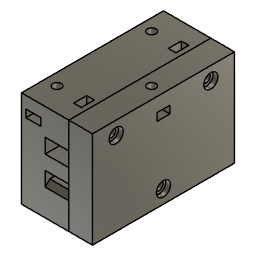
y-belt-holder (Autodesk Fusion 360 design; units mm, degrees)
Autodesk Fusion 360 part; units mm, degrees
sketch "main" plane through (0, 0, 0) normal (1, 0, 0) x (0, 1, 0)
  line L0 (0, 0) -> (60, 0)
  line L1 (60, 0) -> (60, -18.1)
  line L2 (60, -18.1) -> (0, -18.1)
  line L3 (0, -18.1) -> (0, 0)
  line L4 (0, 0) -> (60, 0)
  line L5 (60, 0) -> (60, 17.4)
  line L6 (60, 17.4) -> (0, 17.4)
  line L7 (0, 17.4) -> (0, 0)
  line L8 (0, 17.4) -> (60, 17.4)
  line L9 (60, 17.4) -> (60, 6.15)
  line L10 (60, 6.15) -> (0, 6.15)
  line L11 (0, 6.15) -> (0, 17.4)
  line L12 (0, -18.1) -> (10, -18.1) construction
  line L13 (10, -18.1) -> (10, 0) construction
  line L14 (10, 0) -> (0, 0) construction
  line L15 (0, 0) -> (0, -18.1) construction
  line L16 (60, -18.1) -> (50, -18.1) construction
  line L17 (50, -18.1) -> (50, 0) construction
  line L18 (50, 0) -> (60, 0) construction
  line L19 (60, 0) -> (60, -18.1) construction
  line L20 (10, 0) -> (18, 0)
  line L21 (18, 0) -> (18, -8)
  line L22 (18, -8) -> (10, -8)
  line L23 (10, -8) -> (10, 0)
  line L24 (10, -18.1) -> (18, -18.1)
  line L25 (18, -18.1) -> (18, -10.1)
  line L26 (18, -10.1) -> (10, -10.1)
  line L27 (10, -10.1) -> (10, -18.1)
  line L28 (50, -18.1) -> (42, -18.1)
  line L29 (42, -18.1) -> (42, -10.1)
  line L30 (42, -10.1) -> (50, -10.1)
  line L31 (50, -10.1) -> (50, -18.1)
  line L32 (50, 0) -> (42, 0)
  line L33 (42, 0) -> (42, -8)
  line L34 (42, -8) -> (50, -8)
  line L35 (50, -8) -> (50, 0)
  line L36 (10, 0) -> (18, -8) construction
  line L37 (18, 0) -> (10, -8) construction
  line L38 (42, 0) -> (50, -8) construction
  line L39 (50, 0) -> (42, -8) construction
  line L40 (14, -4) -> (25, -4) construction
  line L41 (46, -4) -> (35, -4) construction
  circle A0 centre (25, -4) radius 4
  circle A1 centre (35, -4) radius 4
  line L42 (0, -10.1) -> (60, -10.1)
  line L43 (0, -8) -> (60, -8)
  dimension "d1" = 60
  dimension "d2" = 18.1
  dimension "d3" = 60
  dimension "d4" = 17.4
  dimension "d5" = 60
  dimension "d6" = 11.25
  dimension "d7" = 10
  dimension "d8" = 18.1
  dimension "d9" = 10
  dimension "d10" = 18.1
  dimension "d11" = 8
  dimension "d12" = 8
  dimension "d13" = 8
  dimension "d14" = 8
  dimension "d15" = 8
  dimension "d16" = 8
  dimension "d17" = 8
  dimension "d18" = 8
  dimension "d19" = 11
  dimension "d20" = 11
  dimension "d21" = 8
  dimension "d22" = 8
  constraint horizontal L0
  constraint vertical L1
  constraint horizontal L2
  constraint vertical L3
  constraint coincident L0.start L3.end
  constraint horizontal L4
  constraint vertical L5
  constraint horizontal L6
  constraint vertical L7
  constraint horizontal L8
  constraint vertical L9
  constraint horizontal L10
  constraint vertical L11
  constraint horizontal L12
  constraint vertical L13
  constraint horizontal L14
  constraint vertical L15
  constraint horizontal L16
  constraint vertical L17
  constraint horizontal L18
  constraint vertical L19
  constraint horizontal L20
  constraint vertical L21
  constraint horizontal L22
  constraint vertical L23
  constraint horizontal L24
  constraint vertical L25
  constraint horizontal L26
  constraint vertical L27
  constraint horizontal L28
  constraint vertical L29
  constraint horizontal L30
  constraint vertical L31
  constraint horizontal L32
  constraint vertical L33
  constraint horizontal L34
  constraint vertical L35
  constraint midpoint L36 L40.start
  constraint perpendicular L21 L40
  constraint midpoint L38 L41.start
  constraint horizontal L41
  constraint coincident L40.end A0.centre
  constraint coincident L41.end A1.centre
  constraint coincident L3 L42.start
  constraint coincident L19 L42.end
  constraint perpendicular L19 L42
  constraint coincident L3 L43.start
  constraint coincident L19 L43.end
  constraint perpendicular L19 L43
  measures "d1" distance of L0.start L0.end
  measures "d2" distance of L0.start L2.end
  measures "d3" distance of L0.start L0.end
  measures "d4" distance of L0.start L6.end
  measures "d5" distance of L6.end L5.end
  measures "d6" distance of L6.end L10.end
  measures "d7" distance of L2.end L12.end
  measures "d8" distance of L2.end L0.start
  measures "d9" distance of L1.end L16.end
  measures "d10" distance of L1.end L0.end
  measures "d11" distance of L13.end L20.end
  measures "d12" distance of L13.end L22.end
  measures "d13" distance of L12.end L24.end
  measures "d14" distance of L12.end L26.end
  measures "d15" distance of L16.end L28.end
  measures "d16" distance of L16.end L30.end
  measures "d17" distance of L17.end L32.end
  measures "d18" distance of L17.end L34.end
  measures "d19" distance of L40.start L40.end
  measures "d20" distance of L41.start L41.end
  measures "d21" diameter of A0
  measures "d22" diameter of A1
extrude "Extrude1" add sketch "main" against normal blind 10 makes body 1
extrude "Extrude2" add sketch "main" along normal blind 10 contours L0 L3 L4 L23 L43 | L0 L4 L20 L21 L22 L23 L43 | L5 L6 L7 L8 L9 L10 L11 | L2 L3 L27 L42 | A0 | L2 L24 L25 L26 L27 L42 | L0 L1 L4 L35 L43 | A1 | L2 L25 L29 L42 | L0 L4 L32 L33 L34 L35 L43 | L2 L28 L29 L30 L31 L42 | L1 L2 L31 L42 bodies 1
chamfer "Chamfer2" distance 2 angle 45 9 edges at (5, 0, -8) (5, 18, -8) (10, 9, -8) (10, 30, -10.1) (5, 0, -10.1) (10, 51, -8) (5, 60, -8) (5, 60, -10.1) (5, 42, -8) on bodies 1
chamfer "Chamfer3" distance 1 angle 45 2 edges at (10, 21.2707, -5.4465) (10, 31.2707, -5.4465) on bodies 1
sketch "main-top-mount" plane through (0, 0, 17.4) normal (0, 0, 1) x (-1, 0, 0)
  line L0 (-10, -60) -> (10, -60)
  line L1 (10, -60) -> (10, 0)
  line L2 (10, 0) -> (-10, 0)
  line L3 (-10, 0) -> (-10, -60)
  line L4 (10, 0) -> (0, 0) construction
  line L5 (0, 0) -> (0, -20) construction
  line L6 (0, -20) -> (10, -20) construction
  line L7 (10, -20) -> (10, 0) construction
  line L8 (10, -60) -> (0, -60) construction
  line L9 (0, -60) -> (0, -40) construction
  line L10 (0, -40) -> (10, -40) construction
  line L11 (10, -40) -> (10, -60) construction
  line L12 (10, 0) -> (0, -20) construction
  line L13 (0, 0) -> (10, -20) construction
  line L14 (10, -60) -> (0, -40) construction
  line L15 (0, -60) -> (10, -40) construction
  circle A0 centre (5, -10) radius 1.8
  circle A1 centre (5, -50) radius 1.8
  line L16 (6.5733, -12.725) -> (8.1466, -10)
  line L17 (8.1466, -10) -> (6.5733, -7.275)
  line L18 (6.5733, -7.275) -> (3.4267, -7.275)
  line L19 (3.4267, -7.275) -> (1.8534, -10)
  line L20 (1.8534, -10) -> (3.4267, -12.725)
  line L21 (3.4267, -12.725) -> (6.5733, -12.725)
  line L22 (6.5733, -52.725) -> (8.1466, -50)
  line L23 (8.1466, -50) -> (6.5733, -47.275)
  line L24 (6.5733, -47.275) -> (3.4267, -47.275)
  line L25 (3.4267, -47.275) -> (1.8534, -50)
  line L26 (1.8534, -50) -> (3.4267, -52.725)
  line L27 (3.4267, -52.725) -> (6.5733, -52.725)
  line L28 (8.1466, -10) -> (8.1466, 0)
  line L29 (1.8534, -10) -> (1.8534, 0)
  line L30 (1.8534, -50) -> (1.8534, -60)
  line L31 (8.1466, -50) -> (8.1466, -60)
  point P0 (5, -10)
  point P1 (5, -50)
  dimension "d32" = 10
  dimension "d33" = 20
  dimension "d34" = 10
  dimension "d35" = 20
  dimension "d36" = 3.6
  dimension "d37" = 3.6
  dimension "d38" = 2.725
  dimension "d39" = 2.725
  dimension "d40" = 10
  dimension "d41" = 10
  dimension "d42" = 10
  dimension "d43" = 10
  constraint horizontal L4
  constraint vertical L5
  constraint horizontal L6
  constraint vertical L7
  constraint coincident L1.end L2.start
  constraint horizontal L8
  constraint vertical L9
  constraint horizontal L10
  constraint vertical L11
  constraint coincident L0.end L1.start
  constraint coincident L4.end L5.start
  constraint midpoint L13 P0
  constraint midpoint L15 P1
  constraint coincident P0 A0.centre
  constraint coincident P1 A1.centre
  constraint vertical L28
  constraint vertical L29
  constraint vertical L30
  constraint vertical L31
  measures "d32" distance of L1.end L4.end
  measures "d33" distance of L1.end L6.end
  measures "d34" distance of L0.end L8.end
  measures "d35" distance of L0.end L10.end
  measures "d36" diameter of A0
  measures "d37" diameter of A1
  measures "d38" distance of P0 L21
  measures "d39" distance of P1 L27
  measures "d40" distance of L16.end L28.end
  measures "d41" distance of L19.end L29.end
  measures "d42" distance of L25.end L30.end
  measures "d43" distance of L22.end L31.end
extrude "Extrude3" cut sketch "main-top-mount" against normal blind 16 contours A0 | A1 bodies 1
extrude "Extrude4" cut sketch "main-top-mount" against normal blind 3.2 from surface at -5 contours L0 L22 L26 L27 L30 L31 | L22 L23 L24 L25 L26 L27 | L2 L17 L18 L19 L28 L29 | L16 L17 L18 L19 L20 L21 bodies 1
extrude "Extrude5" add 1 faces at (3.3333, 40, -18.1) along direction (0, 0, -1) blind 5.25 on bodies 1 bodies 1
sketch "cover" plane through (0, 0, 0) normal (0, 1, 0) x (1, 0, 0)
  line L0 (0, 23.35) -> (10, 23.35) construction
  line L1 (10, 23.35) -> (10, -17.4) construction
  line L2 (10, -17.4) -> (0, -17.4) construction
  line L3 (0, -17.4) -> (0, 23.35) construction
  line L4 (-10, 23.35) -> (10, 23.35) construction
  line L5 (-10, -17.4) -> (10, -17.4) construction
  line L6 (10, 23.35) -> (20, 23.35)
  line L7 (20, 23.35) -> (20, -17.4)
  line L8 (20, -17.4) -> (10, -17.4)
  line L9 (10, -17.4) -> (10, 23.35)
  dimension "d51" = 10
  dimension "d52" = 10
  constraint horizontal L0
  constraint vertical L1
  constraint horizontal L2
  constraint vertical L3
  constraint coincident L1.end L5
  constraint midpoint L0.start L4
  constraint horizontal L6
  constraint vertical L7
  constraint horizontal L8
  constraint vertical L9
  constraint coincident L0.end L1.start
  measures "d51" distance of L0.start L0.end
  measures "d52" distance of L0.end L6.end
extrude "Extrude6" add sketch "cover" along normal blind 60 separate body makes body 2
sketch "cover-joint" plane through (10, 0, 0) normal (1, 0, 0) x (0, 1, 0)
  line L0 (0, 6.15) -> (60, 6.15)
  line L1 (60, 6.15) -> (60, 17.4)
  line L2 (60, 17.4) -> (0, 17.4)
  line L3 (0, 17.4) -> (0, 6.15)
  line L4 (0, 17.4) -> (20, 17.4) construction
  line L5 (20, 17.4) -> (20, 6.15) construction
  line L6 (20, 6.15) -> (0, 6.15) construction
  line L7 (0, 6.15) -> (0, 17.4) construction
  line L8 (60, 17.4) -> (40, 17.4) construction
  line L9 (40, 17.4) -> (40, 6.15) construction
  line L10 (40, 6.15) -> (60, 6.15) construction
  line L11 (60, 6.15) -> (60, 17.4) construction
  line L12 (0, 6.15) -> (60, 6.15) construction
  line L13 (60, 6.15) -> (60, -12.1) construction
  line L14 (60, -12.1) -> (0, -12.1) construction
  line L15 (0, -12.1) -> (0, 6.15) construction
  line L16 (0, -12.1) -> (60, -12.1) construction
  line L17 (60, -12.1) -> (60, -23.35) construction
  line L18 (60, -23.35) -> (0, -23.35) construction
  line L19 (0, -23.35) -> (0, -12.1) construction
  line L20 (0, -12.1) -> (60, -23.35) construction
  line L21 (60, -12.1) -> (0, -23.35) construction
  line L22 (0, 17.4) -> (20, 6.15) construction
  line L23 (20, 17.4) -> (0, 6.15) construction
  line L24 (40, 17.4) -> (60, 6.15) construction
  line L25 (60, 17.4) -> (40, 6.15) construction
  circle A0 centre (10, 11.775) radius 1.8
  circle A1 centre (50, 11.775) radius 1.8
  circle A2 centre (30, -17.725) radius 1.8
  line L26 (32.725, -16.1517) -> (30, -14.5784)
  line L27 (30, -14.5784) -> (27.275, -16.1517)
  line L28 (27.275, -16.1517) -> (27.275, -19.2983)
  line L29 (27.275, -19.2983) -> (30, -20.8716)
  line L30 (30, -20.8716) -> (32.725, -19.2983)
  line L31 (32.725, -19.2983) -> (32.725, -16.1517)
  line L32 (12.725, 13.3483) -> (10, 14.9216)
  line L33 (10, 14.9216) -> (7.275, 13.3483)
  line L34 (7.275, 13.3483) -> (7.275, 10.2017)
  line L35 (7.275, 10.2017) -> (10, 8.6284)
  line L36 (10, 8.6284) -> (12.725, 10.2017)
  line L37 (12.725, 10.2017) -> (12.725, 13.3483)
  line L38 (52.725, 13.3483) -> (50, 14.9216)
  line L39 (50, 14.9216) -> (47.275, 13.3483)
  line L40 (47.275, 13.3483) -> (47.275, 10.2017)
  line L41 (47.275, 10.2017) -> (50, 8.6284)
  line L42 (50, 8.6284) -> (52.725, 10.2017)
  line L43 (52.725, 10.2017) -> (52.725, 13.3483)
  line L44 (7.275, 13.3483) -> (7.275, 17.4)
  line L45 (12.725, 13.3483) -> (12.725, 17.4)
  line L46 (47.275, 13.3483) -> (47.275, 17.4)
  line L47 (52.725, 13.3483) -> (52.725, 17.4)
  line L48 (27.275, -19.2983) -> (27.275, -23.35)
  line L49 (32.725, -19.2983) -> (32.725, -23.35)
  line L50 (27.275, -23.35) -> (32.725, -23.35)
  line L51 (7.275, 17.4) -> (12.725, 17.4)
  line L52 (47.275, 17.4) -> (52.725, 17.4)
  circle A3 centre (10, 11.775) radius 3
  circle A4 centre (50, 11.775) radius 3
  circle A5 centre (30, -17.725) radius 3
  point P0 (30, -17.725)
  point P1 (10, 11.775)
  point P2 (50, 11.775)
  dimension "d55" = 20
  dimension "d56" = 11.25
  dimension "d57" = 20
  dimension "d58" = 11.25
  dimension "d59" = 60
  dimension "d60" = 18.25
  dimension "d61" = 60
  dimension "d62" = 11.25
  dimension "d63" = 3.6
  dimension "d64" = 3.6
  dimension "d65" = 3.6
  dimension "d66" = 2.725
  dimension "d67" = 2.725
  dimension "d68" = 2.725
  dimension "d76" = 6
  dimension "d77" = 6
  dimension "d78" = 6
  constraint horizontal L4
  constraint vertical L5
  constraint horizontal L6
  constraint vertical L7
  constraint coincident L2.end L3.start
  constraint horizontal L8
  constraint vertical L9
  constraint horizontal L10
  constraint vertical L11
  constraint coincident L1.end L2.start
  constraint horizontal L12
  constraint vertical L13
  constraint horizontal L14
  constraint vertical L15
  constraint coincident L0.start L3.end
  constraint horizontal L16
  constraint vertical L17
  constraint horizontal L18
  constraint vertical L19
  constraint midpoint L23 P1
  constraint midpoint L24 P2
  constraint midpoint L20 P0
  constraint coincident P0 A2.centre
  constraint coincident P1 A0.centre
  constraint coincident P2 A1.centre
  constraint vertical L44
  constraint coincident L4 L44.end
  constraint vertical L45
  constraint coincident L4 L45.end
  constraint vertical L46
  constraint coincident L8 L46.end
  constraint vertical L47
  constraint coincident L8 L47.end
  constraint vertical L48
  constraint coincident L18 L48.end
  constraint vertical L49
  constraint coincident L18 L49.end
  constraint concentric A1 A4
  constraint concentric A2 A5
  measures "d55" distance of L2.end L4.end
  measures "d56" distance of L2.end L0.start
  measures "d57" distance of L1.end L8.end
  measures "d58" distance of L1.end L0.end
  measures "d59" distance of L0.start L0.end
  measures "d60" distance of L0.start L14.end
  measures "d61" distance of L14.end L13.end
  measures "d62" distance of L14.end L18.end
  measures "d63" diameter of A0
  measures "d64" diameter of A1
  measures "d65" diameter of A2
  measures "d66" distance of P0 L31
  measures "d67" distance of P1 L37
  measures "d68" distance of P2 L43
  measures "d76" diameter of A3
  measures "d77" diameter of A4
  measures "d78" diameter of A5
extrude "Extrude7" cut sketch "cover-joint" along normal blind 10 and the other way blind 8 contours A0 | A1 | A2 bodies 1 2
extrude "Extrude8" cut sketch "cover-joint" against normal blind 3.2 from surface at -2 contours L2 L32 L33 L44 L45 L51 A3 | L2 L38 L39 L46 L47 L52 A4 | L33 L34 A3 | L38 L43 A4 | L32 L37 A3 | L33 A3 | L32 L33 L34 L35 L36 L37 A3 | L39 L40 A4 | L38 L39 L40 L41 L42 L43 A4 | L38 A4 | L32 A3 | L32 L33 A3 | L34 L35 A3 | L39 A4 | L38 L39 A4 | L42 L43 A4 | L36 L37 A3 | L40 L41 A4 | L35 L36 A3 | L41 L42 A4 | L26 L31 A5 | L26 L27 L28 L29 L30 L31 A5 | L26 L27 A5 | L30 L31 A5 | L29 L30 L48 L49 L50 A5 | L30 A5 | L27 L28 A5 | L29 L30 A5 | L29 A5 | L28 L29 A5 bodies 1
extrude "Extrude9" cut sketch "cover-joint" along normal blind 2 from surface at 8 contours L33 A3 | L32 L33 L34 L35 L36 L37 A3 | L34 A3 | L38 L39 L40 L41 L42 L43 A4 | L38 A4 | L43 A4 | L32 A3 | L37 A3 | L39 A4 | L40 A4 | L35 A3 | L42 A4 | L36 A3 | L41 A4 | L26 L27 L28 L29 L30 L31 A5 | L26 A5 | L31 A5 | L27 A5 | L30 A5 | L28 A5 | L29 A5 bodies 2
sketch "cover-top-mount" plane through (0, 0, 17.4) normal (0, 0, 1) x (-1, 0, 0)
  line L0 (-10, 0) -> (-20, 0)
  line L1 (-20, 0) -> (-20, -60)
  line L2 (-20, -60) -> (-10, -60)
  line L3 (-10, -60) -> (-10, 0)
  line L4 (-10, 0) -> (-20, -60) construction
  line L5 (-10, -60) -> (-20, 0) construction
  circle A0 centre (-15, -30) radius 1.8
  line L6 (-13.4267, -32.725) -> (-11.8534, -30)
  line L7 (-11.8534, -30) -> (-13.4267, -27.275)
  line L8 (-13.4267, -27.275) -> (-16.5733, -27.275)
  line L9 (-16.5733, -27.275) -> (-18.1466, -30)
  line L10 (-18.1466, -30) -> (-16.5733, -32.725)
  line L11 (-16.5733, -32.725) -> (-13.4267, -32.725)
  line L12 (-16.5733, -27.275) -> (-20, -27.275)
  line L13 (-16.5733, -32.725) -> (-20, -32.725)
  line L14 (-20, -32.725) -> (-20, -27.275)
  point P0 (-15, -30)
  dimension "d82" = 3.6
  dimension "d83" = 2.725
  constraint coincident L0.start L3.end
  constraint coincident L1.end L2.start
  constraint coincident L2.end L3.start
  constraint coincident L0.end L1.start
  constraint midpoint L5 P0
  constraint coincident P0 A0.centre
  constraint horizontal L12
  constraint coincident L1 L12.end
  constraint horizontal L13
  constraint coincident L1 L13.end
  measures "d82" diameter of A0
  measures "d83" distance of P0 L11
extrude "Extrude10" cut sketch "cover-top-mount" against normal blind 16 contours A0 bodies 2
extrude "Extrude11" cut sketch "cover-top-mount" against normal blind 3.2 from surface at -5.9 contours L1 L9 L10 L12 L13 L14 | L6 L7 L8 L9 L10 L11 bodies 2
equation "d2 = 8 mm + 8 mm + 2.1 mm"
equation "d4 = 14 mm - ( 18.1 mm - 8 mm ) + 13.5 mm"
equation "d38 = ( 5.45 / 2 ) * 1 mm"
equation "d39 = ( 5.45 / 2 ) * 1 mm"
equation "d66 = ( 5.45 / 2 ) * 1 mm"
equation "d67 = ( 5.45 / 2 ) * 1 mm"
equation "d68 = ( 5.45 / 2 ) * 1 mm"
equation "d83 = ( 5.45 / 2 ) * 1 mm"
equation "d86 = -7.5 mm + 1.6 mm"
named bodies: "y-belt-holder", "cover"
